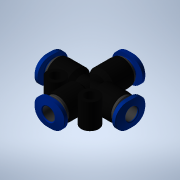
# Autodesk Inventor part: 153379 QSMX-4
Saved by Autodesk Inventor 2021 (Build 250183000, 183)
## iProperties
Created: 2026-09-15
Part Number: 153379 QSMX-4
Material: Generic
Catalog Web Link: www.3dfindit.com
Description: QSMX-Steckverbindung
Vendor: FESTO
Document SubType Name: Modeling
Designer: psAdmin
Manufacturer: FESTO
Mass: 4 g
Surface Area: 24.9685 cm^2
Volume: 1.75764 cm^3
Density: 1 g/cm^3
Appearance: PSOLRGB-176-176-176
Category: PARTsolutions
Company: FESTO
Title: 153379 QSMX-4
Author: Cadenas PARTsolutions
Comments: Steckverbindung
PSOL_IDENT_0: {$CADENAS_DATA/23d-libs/festo/parts/q/qsmx/qsmx.prj},164 {VTYP=3D},{NB=153379 QSMX-4},{LINA=153379 Q
PSOL_IDENT_1: SMX-4},{NN=QSMX},{DATE=05.05.2026 15:29:27},{GEOMDATE=01.04.2025 10:00:42},{VERSION=},{LINEID=20},{W
PSOL_IDENT_2: BVAR=},{WBNUMERIC=}  {NB=153379 QSMX-4},{LINA=153379 QSMX-4},{KT=DUMMY},{TNR=153379},{TYP=QSMX-4},{D
PSOL_IDENT_3: 1=4.000},{NENN=2.500},{D5=8.000},{D6=3.200},{H1=13.500},{H2=5.500},{L1=27.000},{L2=11.000},{CNSMASSE
PSOL_IDENT_4: XACT=0.0040},{L4=11.500},{VERS=1.000},{X=7.800},{Y=9.800},{GTIN=4052568034375},{REACH=Ja},{REACHSVHC=
PSOL_IDENT_5: Ja},{REACHHAZSUBS=7439-92-1},{REACHSCIP=c16a1847-f993-458a-8ccf-4e770ae4a0b5},{REACHVALDATE=05.03.20
PSOL_IDENT_6: 25}
NB: 153379 QSMX-4
NN: QSMX
NT: Steckverbindung
NBSYN: $TNR. $TYP.
LINA: 153379 QSMX-4
CATALOG: Festo
TNR: 153379
TYP: QSMX-4
D1: 4
NENN: 2.5
D5: 8
D6: 3.2
H1: 13.5
H2: 5.5
L1: 27
L2: 11
CNSMASSEXACT: 0.004
GTIN: 4052568034375
REACH: Yes
REACHSVHC: Yes
REACHHAZSUBS: 7439-92-1
REACHVALDATE: 05.03.2025
SUPPLIER: FESTO
ARTICLENO: 153379 QSMX-4
BOMINFO: 153379 QSMX-4
CREATOR: CADENAS GmbH
Autodesk Inventor part; units mm, degrees
sketch "Sketch_1" plane through (0, 0, 0) normal (0, 1, 0) x (-1, 0, 0)
  line L0 (-13.5, 0) -> (13.5, 0)
  line L1 (13.5, 0) -> (13.5, -2.3)
  line L2 (13.5, -2.3) -> (13.0707, -4.7347)
  arc A0 (12.8737, -4.9) -> (13.0707, -4.7347) centre (12.8737, -4.7) ccw
  line L3 (12.8737, -4.9) -> (12, -4.9)
  line L4 (12, -4.9) -> (12, -3)
  arc A1 (12, -3) -> (11.7, -2.7) centre (11.7, -3) ccw
  line L5 (11.7, -2.7) -> (11.2, -2.7)
  line L6 (11.2, -2.7) -> (11.2, -3.4586)
  line L7 (11.2, -3.4586) -> (11.0586, -3.6)
  line L8 (11.0586, -3.6) -> (10.4, -3.6)
  line L9 (10.4, -3.6) -> (10.4, -3.8949)
  line L10 (10.4, -3.8949) -> (9.4, -4)
  line L11 (9.4, -4) -> (4, -4)
  line L12 (4, -4) -> (2.8, -2.8)
  line L13 (2.8, -2.8) -> (-2.8, -2.8)
  line L14 (-2.8, -2.8) -> (-4, -4)
  line L15 (-4, -4) -> (-9.4, -4)
  line L16 (-9.4, -4) -> (-10.4, -3.8949)
  line L17 (-10.4, -3.8949) -> (-10.4, -3.6)
  line L18 (-10.4, -3.6) -> (-11.0586, -3.6)
  line L19 (-11.0586, -3.6) -> (-11.2, -3.4586)
  line L20 (-11.2, -3.4586) -> (-11.2, -2.7)
  line L21 (-11.2, -2.7) -> (-11.7, -2.7)
  arc A2 (-11.7, -2.7) -> (-12, -3) centre (-11.7, -3) ccw
  line L22 (-12, -3) -> (-12, -4.9)
  line L23 (-12, -4.9) -> (-12.7898, -4.9)
  arc A3 (-13.0853, -4.6521) -> (-12.7898, -4.9) centre (-12.7898, -4.6) ccw
  line L24 (-13.0853, -4.6521) -> (-13.5, -2.3)
  line L25 (-13.5, -2.3) -> (-13.5, 0)
  line L26 (-13.5, 0) -> (13.5, 0)
  constraints: 54 end point, 8 point on circle, 4 centre point
revolve "Revolution1" add sketch "Sketch_1" angle 360 about axis through (13.5, 0, 0) along (1, 0, 0)
sketch "Sketch_4" plane through (0, 0, 0) normal (0, 1, 0) x (-1, 0, 0)
  line L0 (0, -13.5) -> (0, 13.5)
  line L1 (0, 13.5) -> (2.3, 13.5)
  line L2 (2.3, 13.5) -> (4.7347, 13.0707)
  arc A0 (4.9, 12.8737) -> (4.7347, 13.0707) centre (4.7, 12.8737) ccw
  line L3 (4.9, 12.8737) -> (4.9, 12)
  line L4 (4.9, 12) -> (3, 12)
  arc A1 (3, 12) -> (2.7, 11.7) centre (3, 11.7) ccw
  line L5 (2.7, 11.7) -> (2.7, 11.2)
  line L6 (2.7, 11.2) -> (3.4586, 11.2)
  line L7 (3.4586, 11.2) -> (3.6, 11.0586)
  line L8 (3.6, 11.0586) -> (3.6, 10.4)
  line L9 (3.6, 10.4) -> (3.8949, 10.4)
  line L10 (3.8949, 10.4) -> (4, 9.4)
  line L11 (4, 9.4) -> (4, 3.85)
  line L12 (4, 3.85) -> (2.8, 2.65)
  line L13 (2.8, 2.65) -> (2.8, -2.65)
  line L14 (2.8, -2.65) -> (4, -3.85)
  line L15 (4, -3.85) -> (4, -9.4)
  line L16 (4, -9.4) -> (3.8949, -10.4)
  line L17 (3.8949, -10.4) -> (3.6, -10.4)
  line L18 (3.6, -10.4) -> (3.6, -11.0586)
  line L19 (3.6, -11.0586) -> (3.4586, -11.2)
  line L20 (3.4586, -11.2) -> (2.7, -11.2)
  line L21 (2.7, -11.2) -> (2.7, -11.7)
  arc A2 (2.7, -11.7) -> (3, -12) centre (3, -11.7) ccw
  line L22 (3, -12) -> (4.9, -12)
  line L23 (4.9, -12) -> (4.9, -12.7898)
  arc A3 (4.6521, -13.0853) -> (4.9, -12.7898) centre (4.6, -12.7898) ccw
  line L24 (4.6521, -13.0853) -> (2.3, -13.5)
  line L25 (2.3, -13.5) -> (0, -13.5)
  line L26 (0, -13.5) -> (0, 13.5)
  constraints: 54 end point, 8 point on circle, 4 centre point
revolve "Revolution2" add sketch "Sketch_4" angle 360 about axis through (0, 0, -13.5) along (0, 0, -1)
sketch "Sketch_11" plane through (0, 0, 5.5) normal (0, 0, 1) x (1, 0, 0)
  line L0 (-5.5, 4) -> (-5.5, -4)
  line L1 (-5.5, -4) -> (-8.3, -4)
  line L2 (-8.3, -4) -> (-8.3, 4)
  line L3 (-8.3, 4) -> (-5.5, 4)
  line L4 (-5.5, 4) -> (-5.5, -4)
  constraints: 10 end point
revolve "Revolution3" add sketch "Sketch_11" angle 360 about axis through (-5.5, 4, 5.5) along (0, 1, 0)
sketch "Sketch_12" plane through (0, 0, 5.5) normal (0, 0, 1) x (1, 0, 0)
  line L0 (5.5, 4) -> (5.5, -4)
  line L1 (5.5, -4) -> (2.7, -4)
  line L2 (2.7, -4) -> (2.7, 4)
  line L3 (2.7, 4) -> (5.5, 4)
  line L4 (5.5, 4) -> (5.5, -4)
  constraints: 10 end point
revolve "Revolution4" add sketch "Sketch_12" angle 360 about axis through (5.5, 4, 5.5) along (0, 1, 0)
sketch "Sketch5" plane through (-5.5, 4, 5.5) normal (0, 1, 0) x (1, 0, 0)
  point P0 (0, 0)
hole "Hole1" at (-5.5, 4, 5.5) direction (0, -1, 0) diameter 3.2 depth 8
sketch "Sketch6" plane through (5.5, 4, 5.5) normal (0, 1, 0) x (1, 0, 0)
  point P0 (0, 0)
hole "Hole2" at (5.5, 4, 5.5) direction (0, -1, 0) diameter 3.2 depth 8
sketch "Sketch_2" plane through (13.5, 0, 0) normal (1, 0, 0) x (0, 0, -1)
  line L0 (-5.88, -5.88) -> (5.88, -5.88)
  line L1 (5.88, -5.88) -> (5.88, 5.88)
  line L2 (5.88, 5.88) -> (-5.88, 5.88)
  line L3 (-5.88, 5.88) -> (-5.88, -5.88)
  arc A0 (-1, 3.9) -> (-1, -3.9) centre (-1, 0) ccw
  line L4 (-1, -3.9) -> (1, -3.9)
  arc A1 (1, -3.9) -> (1, 3.9) centre (1, 0) ccw
  line L5 (1, 3.9) -> (-1, 3.9)
  constraints: 12 end point, 4 point on circle, 2 centre point
extrude "Extrusion1" cut sketch "Sketch_2" against normal blind 1.5
sketch "Sketch_6" plane through (-13.5, 0, 0) normal (1, 0, 0) x (0, 0, -1)
  line L0 (-5.88, -5.88) -> (5.88, -5.88)
  line L1 (5.88, -5.88) -> (5.88, 5.88)
  line L2 (5.88, 5.88) -> (-5.88, 5.88)
  line L3 (-5.88, 5.88) -> (-5.88, -5.88)
  arc A0 (-1, 3.9) -> (-1, -3.9) centre (-1, 0) ccw
  line L4 (-1, -3.9) -> (1, -3.9)
  arc A1 (1, -3.9) -> (1, 3.9) centre (1, 0) ccw
  line L5 (1, 3.9) -> (-1, 3.9)
  constraints: 12 end point, 4 point on circle, 2 centre point
extrude "Extrusion2" cut sketch "Sketch_6" along normal blind 1.5
sketch "Sketch_8" plane through (0, 0, 13.5) normal (0, 0, 1) x (1, 0, 0)
  line L0 (-5.88, -5.88) -> (5.88, -5.88)
  line L1 (5.88, -5.88) -> (5.88, 5.88)
  line L2 (5.88, 5.88) -> (-5.88, 5.88)
  line L3 (-5.88, 5.88) -> (-5.88, -5.88)
  arc A0 (-1, 3.9) -> (-1, -3.9) centre (-1, 0) ccw
  line L4 (-1, -3.9) -> (1, -3.9)
  arc A1 (1, -3.9) -> (1, 3.9) centre (1, 0) ccw
  line L5 (1, 3.9) -> (-1, 3.9)
  constraints: 12 end point, 4 point on circle, 2 centre point
extrude "Extrusion3" cut sketch "Sketch_8" against normal blind 1.5
sketch "Sketch_9" plane through (0, 0, -13.5) normal (0, 0, 1) x (1, 0, 0)
  line L0 (-5.88, -5.88) -> (5.88, -5.88)
  line L1 (5.88, -5.88) -> (5.88, 5.88)
  line L2 (5.88, 5.88) -> (-5.88, 5.88)
  line L3 (-5.88, 5.88) -> (-5.88, -5.88)
  arc A0 (-1, 3.9) -> (-1, -3.9) centre (-1, 0) ccw
  line L4 (-1, -3.9) -> (1, -3.9)
  arc A1 (1, -3.9) -> (1, 3.9) centre (1, 0) ccw
  line L5 (1, 3.9) -> (-1, 3.9)
  constraints: 12 end point, 4 point on circle, 2 centre point
extrude "Extrusion4" cut sketch "Sketch_9" along normal blind 1.5
sketch "Sketch_7" plane through (0, 0, 0) normal (0, 0, 1) x (1, 0, 0)
  line L0 (13.5, 0) -> (-13.5, 0)
  line L1 (-13.5, 0) -> (-13.5, 2.3)
  arc A0 (-13.5, 2.3) -> (-13.2, 2) centre (-13.2, 2.3) ccw
  line L2 (-13.2, 2) -> (-2.1, 2)
  arc A1 (-2, 1.9) -> (-2.1, 2) centre (-2.1, 1.9) ccw
  line L3 (-2, 1.9) -> (-2, 1.25)
  line L4 (-2, 1.25) -> (2, 1.25)
  line L5 (2, 1.25) -> (2, 1.9)
  arc A2 (2.1, 2) -> (2, 1.9) centre (2.1, 1.9) ccw
  line L6 (2.1, 2) -> (13.2, 2)
  arc A3 (13.2, 2) -> (13.5, 2.3) centre (13.2, 2.3) ccw
  line L7 (13.5, 2.3) -> (13.5, 0)
  line L8 (13.5, 0) -> (-13.5, 0)
  constraints: 18 end point, 8 point on circle, 4 centre point
revolve "Revolution5" cut sketch "Sketch_7" angle 360 about axis through (13.5, 0, 0) along (1, 0, 0)
sketch "Sketch_10" plane through (0, 0, 0) normal (1, 0, 0) x (0, 1, 0)
  line L0 (0, -13.5) -> (0, 13.5)
  line L1 (0, 13.5) -> (2.3, 13.5)
  arc A0 (2.3, 13.5) -> (2, 13.2) centre (2.3, 13.2) ccw
  line L2 (2, 13.2) -> (2, 2.1)
  arc A1 (1.9, 2) -> (2, 2.1) centre (1.9, 2.1) ccw
  line L3 (1.9, 2) -> (1.45, 2)
  line L4 (1.45, 2) -> (1.45, -2)
  line L5 (1.45, -2) -> (1.9, -2)
  arc A2 (2, -2.1) -> (1.9, -2) centre (1.9, -2.1) ccw
  line L6 (2, -2.1) -> (2, -13.2)
  arc A3 (2, -13.2) -> (2.3, -13.5) centre (2.3, -13.2) ccw
  line L7 (2.3, -13.5) -> (0, -13.5)
  line L8 (0, -13.5) -> (0, 13.5)
  constraints: 18 end point, 8 point on circle, 4 centre point
revolve "Revolution6" cut sketch "Sketch_10" angle 360 about axis through (0, 0, -13.5) along (0, 0, -1)
ref_plane "ANBAU_XY" through (0, 0, -13.5) normal (0, 0, 1) x (1, 0, 0)
ref_plane "ANBAU_YZ" through (0, 0, -13.5) normal (1, 0, 0) x (0, 1, 0)
ref_plane "ANBAU_ZX" through (0, 0, -13.5) normal (0, 1, 0) x (0, 0, 1)
ref_plane "CP1_XY" through (13.5, 0, 0) normal (-1, 0, 0) x (0, 0, -1)
ref_plane "CP1_YZ" through (13.5, 0, 0) normal (0, 0, -1) x (0, -1, 0)
ref_plane "CP1_ZX" through (13.5, 0, 0) normal (0, -1, 0) x (-1, 0, 0)
ref_plane "CP2_XY" through (-13.5, 0, 0) normal (1, 0, 0) x (0, 0, -1)
ref_plane "CP2_YZ" through (-13.5, 0, 0) normal (0, 0, -1) x (0, 1, 0)
ref_plane "CP2_ZX" through (-13.5, 0, 0) normal (0, 1, 0) x (1, 0, 0)
ref_plane "CP3_XY" through (0, 0, 13.5) normal (0, 0, -1) x (1, 0, 0)
ref_plane "CP3_YZ" through (0, 0, 13.5) normal (1, 0, 0) x (0, -1, 0)
ref_plane "CP3_ZX" through (0, 0, 13.5) normal (0, -1, 0) x (0, 0, -1)
body "Solid1"
